Autodesk Fusion 360 part; units mm, degrees
(part 7 of 7)
  spline S47 degree 3 poles (-28.9778, 7.7644) (-29.036, 7.5424) (-29.0052, 7.3365) (-28.9606, 7.2236) (-28.942, 7.1764) (-28.9203, 7.1406) (-28.9025, 7.1161) (-28.8924, 7.1022) (-28.884, 7.0919) (-28.8332, 7.031) (-28.8015, 6.993) (-28.7553, 6.947) (-28.6638, 6.8038) (-28.5987, 6.7019) (-28.4905, 6.5146) (-28.4393, 6.242) (-28.3991, 6.0278) (-28.4161, 5.8162) (-28.4329, 5.7122) (-28.4484, 5.6167) (-28.4607, 5.5388) (-28.5278, 5.3746) (-28.6119, 5.1689) (-28.789, 4.9345) (-28.9196, 4.8156) (-29.1619, 4.5951) (-29.2503, 4.5799) (-29.3108, 4.5478) (-29.445, 4.4767) (-29.4238, 4.4889) (-29.4531, 4.4677) (-29.5491, 4.3982) (-29.7033, 4.2078) (-29.7434, 3.9157) knots 0.001251 0.001251 0.001251 0.001251 0.25 0.25 0.25 0.35404 0.35404 0.35404 0.412746 0.412746 0.412746 0.449449 0.449449 0.449449 0.475576 0.475576 0.475576 0.496118 0.496118 0.496118 0.514995 0.514995 0.514995 0.538647 0.538647 0.538647 0.582499 0.582499 0.582499 0.679826 0.679826 0.679826 0.99875 0.99875 0.99875 0.99875
  dimension "d71" = 1.5
  dimension "d72" = -1.5
  dimension "d74" = 360
  dimension "d75" = 30
  dimension "d76" = 1.5
  dimension "d77" = -1.5
  dimension "d78" = 60
  dimension "d79" = -3
  dimension "d80" = 3
  dimension "d82" = 360
  constraint coincident A3.centre L0.start
  constraint concentric A6 A9
  measures "d75" diameter of A6
  measures "d78" diameter of A9
extrude "Extrude3" cut sketch "Sketch3" against normal blind 6 contours L5 L8 A7 A10 A13 A14 | L3 L6 A7 A10 A12 A13 | L2 L4 A7 A10 A11 A12 | L7 L10 A7 A10 A14 A15 | L1 L9 A7 A10 A11 A15
fillet "Fillet2" radius 3 30 edges at (9.7572, -25.1753, 1.2) (8.4902, -21.2758, 1.2) (12.0526, -11.2687, 1.2) (14.4417, -7.9805, 1.2) (22.8581, -1.4999, 1.2) (26.9583, -1.4999, 1.2) (6.9041, -26.1024, 1.2) (5.637, -22.2029, 1.2) (-3.1272, -16.2009, 1.2) (-6.9927, -14.945, 1.2) (-17.6109, -14.6492, 1.2) (-20.928, -17.0593, 1.2) (-22.6914, -14.6322, 1.2) (-19.3742, -12.2222, 1.2) (-16.3744, -2.0322, 1.2) (-16.3744, 2.0322, 1.2) (-19.3743, 12.2221, 1.2) (-22.6915, 14.6321, 1.2) (-20.9281, 17.0591, 1.2) (-17.611, 14.6491, 1.2) (-6.9927, 14.945, 1.2) (-3.1272, 16.2009, 1.2) (5.6369, 22.2029, 1.2) (6.9039, 26.1024, 1.2) (9.7571, 25.1754, 1.2) (8.4901, 21.2759, 1.2) (12.0526, 11.2687, 1.2) (14.4417, 7.9805, 1.2) (22.8581, 1.5001, 1.2) (26.9583, 1.5001, 1.2)
mirror "Mirror1" about plane through (0, 0, 0) normal (0, 0, -1) of bodies 1 merged
equation "d1 = ( 30.367 * 2 ) * 1 mm"
equation "d2 = ( 0.633 * 2 ) * 1 mm"
equation "d22 = ( 49 * 0.5 ) * 1 deg"
equation "d27 = ( 49 * 1.5 ) * 1 deg"
equation "d29 = ( 49 * 2 ) * 1 deg"
equation "d32 = ( 49 * 2.5 ) * 1 deg"
equation "d33 = ( 49 * 3 ) * 1 deg"
equation "d35 = ( 49 * 3.5 ) * 1 deg"
equation "d56 = ( 7.5 * 49 ) * 1 deg"

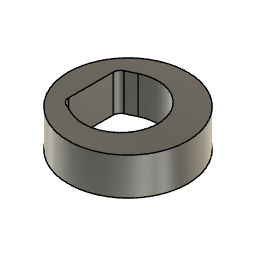
design "eccentric nut"
Autodesk Fusion 360 part; units mm, degrees
sketch "Sketch1" plane through (0, 0, 0) normal (0, 0, 1) x (1, 0, 0)
  circle A0 centre (0, 0) radius 4
  circle A1 centre (-0.5, 0) radius 2.5
  line L0 (-2.5, 1.5) -> (-2.5, -1.5)
  circle A2 centre (-2, 1.5) radius 0.5
  line L1 (-2.8087, 1.6679) -> (-0.6979, 2.676)
  line L2 (-0.5, 0) -> (0, 0)
  line L3 (-2.8087, -1.6679) -> (-0.6979, -2.676)
  circle A3 centre (-2, -1.5) radius 0.5
  dimension "d1" = 8
  dimension "d2" = 5
  dimension "d3" = 0.5
  dimension "d4" = 2
  dimension "d13" = 1
  constraint coincident A0.centre L2.end
  constraint horizontal A0.centre A1.centre
  constraint vertical L0
  constraint coincident A1 L0.start
  constraint coincident A1 L0.end
  constraint horizontal A2.centre L0.start
  constraint tangent L0 A2
  constraint tangent A1 L1
  constraint tangent A2 L1
  constraint coincident A1.centre L2.start
  constraint symmetric A2 L2 A3
  constraint symmetric L1.start L2 L3.start
  constraint symmetric L1.end L2 L3.end
  measures "d1" diameter of A0
  measures "d2" diameter of A1
  measures "d3" distance of A0.centre A1.centre
  measures "d4" distance of A1.centre L0
  measures "d13" diameter of A2
extrude "Extrude3" add sketch "Sketch1" along normal blind 2.5 contours A0 | A1 L0

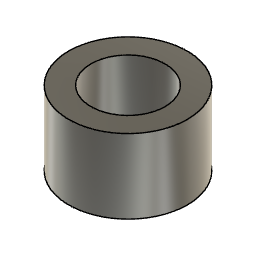
design "nylon spacer"
Autodesk Fusion 360 part; units mm, degrees
sketch "Sketch1" plane through (0, 0, 0) normal (0, 0, 1) x (1, 0, 0)
  circle A0 centre (0, 0) radius 4
  circle A1 centre (0, 0) radius 2.5
  dimension "d1" = 8
  dimension "d2" = 5
  constraint coincident A0.centre A1.centre
  constraint concentric A0 A1
  measures "d1" diameter of A0
  measures "d2" diameter of A1
extrude "Extrude1" add sketch "Sketch1" along normal blind 5

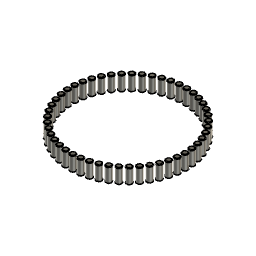
design "cylindrical pins"
Autodesk Fusion 360 part; units mm, degrees
sketch "Sketch1" plane through (0, 0, 0) normal (0, 0, 1) x (1, 0, 0)
  circle A0 centre (31, 0) radius 1.5
  dimension "d1" = 3
  dimension "d2" = 31
  constraint horizontal origin A0.centre
  measures "d1" diameter of A0
  measures "d2" distance of origin A0.centre
extrude "Extrude1" add sketch "Sketch1" along normal blind 8 makes body 1
chamfer "Chamfer1" distance 0.3 angle 45 2 edges at (29.6015, -0.5424, 8) (29.6015, -0.5424, 0) on bodies 1
pattern_circular "C-Pattern1" count 49 over 360 about axis through (0, 0, 1.75) along (0, 0, 1) of bodies 1 makes body 2 at (32.2449, 4.0069, 5.2333) makes body 3 at (31.4678, 8.0974, 5.2333) makes body 4 at (30.1739, 12.0549, 5.2333) makes body 5 at (28.3847, 15.8145, 5.2333) makes body 6 at (26.1293, 19.3144, 5.2333) makes body 7 at (23.4449, 22.4972, 5.2333) makes body 8 at (18.7113, 22.8695, 5.2333) makes body 9 at (16.9716, 27.7083, 5.2333) makes body 10 at (13.289, 29.6511, 5.2333) makes body 11 at (9.3882, 31.1071, 5.2333) makes body 12 at (5.3332, 32.0522, 5.2333) makes body 13 at (1.1907, 32.4711, 5.2333) makes body 14 at (-2.9714, 32.3567, 5.2333) makes body 15 at (-7.0847, 31.7111, 5.2333) makes body 16 at (-11.0816, 30.5448, 5.2333) makes body 17 at (-14.8966, 28.8769, 5.2333) makes body 18 at (-18.467, 26.7349, 5.2333) makes body 19 at (-22.3412, 22.9272, 5.2333) makes body 20 at (-24.6445, 21.1763, 5.2333) makes body 21 at (-25.6888, 15.4403, 5.2333) makes body 22 at (-29.21, 14.2325, 5.2333) makes body 23 at (-30.7902, 10.3804, 5.2333) makes body 24 at (-31.8648, 6.3578, 5.2333) makes body 25 at (-32.4162, 2.2308, 5.2333) makes body 26 at (-32.4354, -1.9328, 5.2333) makes body 27 at (-31.9219, -6.0646, 5.2333) makes body 28 at (-30.8843, -10.0969, 5.2333) makes body 29 at (-29.3396, -13.9634, 5.2333) makes body 30 at (-25.6888, -15.4403, 5.2333) makes body 31 at (-24.8381, -20.9489, 5.2333) makes body 32 at (-21.9553, -23.9531, 5.2333) makes body 33 at (-18.712, -26.564, 5.2333) makes body 34 at (-15.1615, -28.7388, 5.2333) makes body 35 at (-11.2939, -30.4727, 5.2333) makes body 36 at (-7.3044, -31.6667, 5.2333) makes body 37 at (-1.5824, -30.3038, 5.2333) makes body 38 at (0.8922, -32.4806, 5.2333) makes body 39 at (5.0384, -32.0999, 5.2333) makes body 40 at (9.1018, -31.1921, 5.2333) makes body 41 at (13.0159, -29.772, 5.2333) makes body 42 at (16.9107, -27.7518, 2.7667) makes body 43 at (20.2038, -25.4547, 5.2333) makes body 44 at (23.2371, -22.7118, 5.2333) makes body 45 at (26.2302, -19.1142, 5.2333) makes body 46 at (28.2381, -16.0748, 5.2333) makes body 47 at (30.095, -12.2648, 5.2333) makes body 48 at (31.392, -8.3864, 5.2333) makes body 49 at (30.2983, -5.396, 2.7667)
equation "d2 = ( 62 / 2 ) * 1 mm"

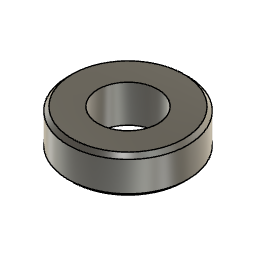
design "16x8x5 bearing"
Autodesk Fusion 360 part; units mm, degrees
sketch "Sketch1" plane through (0, 0, 0) normal (0, 0, 1) x (1, 0, 0)
  circle A0 centre (0, 0) radius 8
  circle A1 centre (0, 0) radius 4
  dimension "d1" = 16
  dimension "d2" = 8
  constraint coincident A0.centre A1.centre
  measures "d1" diameter of A0
  measures "d2" diameter of A1
extrude "Extrude1" add sketch "Sketch1" along normal blind 5
chamfer "Chamfer1" distance 0.5 angle 45 2 edges at (-7.4586, -2.8929, 5) (-7.4586, -2.8929, 0)

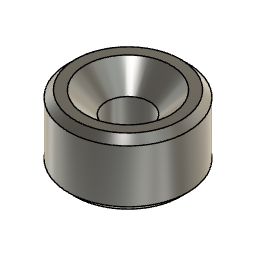
design "torque output pins"
Autodesk Fusion 360 part; units mm, degrees
sketch "Sketch1" plane through (0, 0, 0) normal (0, 0, 1) x (1, 0, 0)
  circle A0 centre (0, 0) radius 4.5
  circle A1 centre (0, 0) radius 1.5
  dimension "d1" = 9
  dimension "d4" = 3
  constraint coincident A0.centre A1.centre
  measures "d1" diameter of A0
  measures "d4" diameter of A1
extrude "Extrude1" add sketch "Sketch1" along normal blind 5
hole "Hole1" at (0, 0, 5) direction (0, 0, -1) diameter 3.3 depth 10 tip angle 118 countersink diameter 6.5 countersink angle 90
chamfer "Chamfer1" distance 0.5 angle 45 2 edges at (-4.1955, -1.6273, 5) (-4.1955, -1.6273, 0)
